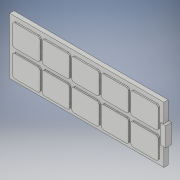
# Autodesk Inventor part: Solar_panel
Saved by Autodesk Inventor 2018 (Build 220112000, 112)
## iProperties
Created: 2021-03-12
Part Number: Solar_panel
Material: Generic
Document SubType Name: Modeling
Designer: Patel
Density: 1 g/cm^3
Appearance: Default
Author: Patel
Autodesk Inventor part; units mm, degrees
ref_plane "YZ Plane" through (0, 0, 0) normal (1, 0, 0) x (0, 1, 0)
ref_plane "XZ Plane" through (0, 0, 0) normal (0, 1, 0) x (-1, 0, 0)
sketch "Sketch1" plane through (0, 0, 0) normal (0, 0, 1) x (1, 0, 0)
  line L0 (-177.5, 65) -> (177.5, 65)
  line L1 (177.5, 65) -> (177.5, -65)
  line L2 (177.5, -65) -> (-177.5, -65)
  line L3 (-177.5, -65) -> (-177.5, 65)
  line L4 (-177.5, 65) -> (177.5, -65) construction
  line L5 (177.5, 65) -> (-177.5, -65) construction
  point P0 (0, 0)
  dimension "d0" = 355
  dimension "d1" = 130
  constraints: 12 end point, 2 midpoint, 2 parallel, 1 horizontal, 1 perpendicular
  measures "d0" distance of L1.end L2.end
  measures "d1" distance of L0.end L1.end
extrude "Extrusion1" add sketch "Sketch1" against normal blind 10
sketch "Sketch2" plane through (0, 0, 0) normal (0, 0, 1) x (1, 0, 0)
  line L0 (-162.5, 55) -> (-109.5, 55)
  line L1 (-104.5, 50) -> (-104.5, 9.1977)
  line L2 (-109.5, 4.1977) -> (-162.5, 4.1977)
  line L3 (-167.5, 9.1977) -> (-167.5, 50)
  line L4 (-177.5, 65) -> (177.5, 65) projected
  line L5 (-177.5, -65) -> (-177.5, 65) projected
  arc A0 (-162.5, 55) -> (-167.5, 50) centre (-162.5, 50) ccw
  arc A1 (-104.5, 50) -> (-109.5, 55) centre (-109.5, 50) ccw
  arc A2 (-109.5, 4.1977) -> (-104.5, 9.1977) centre (-109.5, 9.1977) ccw
  arc A3 (-167.5, 9.1977) -> (-162.5, 4.1977) centre (-162.5, 9.1977) ccw
  line L6 (-94.5, 55) -> (-41.5, 55)
  line L7 (-36.5, 50) -> (-36.5, 9.1977)
  line L8 (-41.5, 4.1977) -> (-94.5, 4.1977)
  line L9 (-99.5, 9.1977) -> (-99.5, 50)
  arc A4 (-94.5, 55) -> (-99.5, 50) centre (-94.5, 50) ccw
  arc A5 (-36.5, 50) -> (-41.5, 55) centre (-41.5, 50) ccw
  arc A6 (-41.5, 4.1977) -> (-36.5, 9.1977) centre (-41.5, 9.1977) ccw
  arc A7 (-99.5, 9.1977) -> (-94.5, 4.1977) centre (-94.5, 9.1977) ccw
  line L10 (-26.5, 55) -> (26.5, 55)
  line L11 (31.5, 50) -> (31.5, 9.1977)
  line L12 (26.5, 4.1977) -> (-26.5, 4.1977)
  line L13 (-31.5, 9.1977) -> (-31.5, 50)
  arc A8 (-26.5, 55) -> (-31.5, 50) centre (-26.5, 50) ccw
  arc A9 (31.5, 50) -> (26.5, 55) centre (26.5, 50) ccw
  arc A10 (26.5, 4.1977) -> (31.5, 9.1977) centre (26.5, 9.1977) ccw
  arc A11 (-31.5, 9.1977) -> (-26.5, 4.1977) centre (-26.5, 9.1977) ccw
  line L14 (41.5, 55) -> (94.5, 55)
  line L15 (99.5, 50) -> (99.5, 9.1977)
  line L16 (94.5, 4.1977) -> (41.5, 4.1977)
  line L17 (36.5, 9.1977) -> (36.5, 50)
  arc A12 (41.5, 55) -> (36.5, 50) centre (41.5, 50) ccw
  arc A13 (99.5, 50) -> (94.5, 55) centre (94.5, 50) ccw
  arc A14 (94.5, 4.1977) -> (99.5, 9.1977) centre (94.5, 9.1977) ccw
  arc A15 (36.5, 9.1977) -> (41.5, 4.1977) centre (41.5, 9.1977) ccw
  line L18 (109.5, 55) -> (162.5, 55)
  line L19 (167.5, 50) -> (167.5, 9.1977)
  line L20 (162.5, 4.1977) -> (109.5, 4.1977)
  line L21 (104.5, 9.1977) -> (104.5, 50)
  arc A16 (109.5, 55) -> (104.5, 50) centre (109.5, 50) ccw
  arc A17 (167.5, 50) -> (162.5, 55) centre (162.5, 50) ccw
  arc A18 (162.5, 4.1977) -> (167.5, 9.1977) centre (162.5, 9.1977) ccw
  arc A19 (104.5, 9.1977) -> (109.5, 4.1977) centre (109.5, 9.1977) ccw
  line L22 (-162.5, -5.802) -> (-109.5, -5.802)
  line L23 (-167.5, -51.6043) -> (-167.5, -10.802)
  line L24 (-109.5, -56.6043) -> (-162.5, -56.6043)
  line L25 (-104.5, -10.802) -> (-104.5, -51.6043)
  line L26 (-99.5, -51.6043) -> (-99.5, -10.802)
  line L27 (-94.5, -5.802) -> (-41.5, -5.802)
  line L28 (-36.5, -10.802) -> (-36.5, -51.6043)
  line L29 (-41.5, -56.6043) -> (-94.5, -56.6043)
  line L30 (-31.5, -51.6043) -> (-31.5, -10.802)
  line L31 (-26.5, -5.802) -> (26.5, -5.802)
  line L32 (31.5, -10.802) -> (31.5, -51.6043)
  line L33 (26.5, -56.6043) -> (-26.5, -56.6043)
  line L34 (41.5, -5.802) -> (94.5, -5.802)
  line L35 (36.5, -51.6043) -> (36.5, -10.802)
  line L36 (94.5, -56.6043) -> (41.5, -56.6043)
  line L37 (99.5, -10.802) -> (99.5, -51.6043)
  line L38 (104.5, -51.6043) -> (104.5, -10.802)
  line L39 (109.5, -5.802) -> (162.5, -5.802)
  line L40 (167.5, -10.802) -> (167.5, -51.6043)
  line L41 (162.5, -56.6043) -> (109.5, -56.6043)
  arc A20 (-162.5, -5.802) -> (-167.5, -10.802) centre (-162.5, -10.802) ccw
  arc A21 (-104.5, -10.802) -> (-109.5, -5.802) centre (-109.5, -10.802) ccw
  arc A22 (-167.5, -51.6043) -> (-162.5, -56.6043) centre (-162.5, -51.6043) ccw
  arc A23 (-109.5, -56.6043) -> (-104.5, -51.6043) centre (-109.5, -51.6043) ccw
  arc A24 (-99.5, -51.6043) -> (-94.5, -56.6043) centre (-94.5, -51.6043) ccw
  arc A25 (-94.5, -5.802) -> (-99.5, -10.802) centre (-94.5, -10.802) ccw
  arc A26 (-36.5, -10.802) -> (-41.5, -5.802) centre (-41.5, -10.802) ccw
  arc A27 (-26.5, -5.802) -> (-31.5, -10.802) centre (-26.5, -10.802) ccw
  arc A28 (-41.5, -56.6043) -> (-36.5, -51.6043) centre (-41.5, -51.6043) ccw
  arc A29 (-31.5, -51.6043) -> (-26.5, -56.6043) centre (-26.5, -51.6043) ccw
  arc A30 (31.5, -10.802) -> (26.5, -5.802) centre (26.5, -10.802) ccw
  arc A31 (26.5, -56.6043) -> (31.5, -51.6043) centre (26.5, -51.6043) ccw
  arc A32 (36.5, -51.6043) -> (41.5, -56.6043) centre (41.5, -51.6043) ccw
  arc A33 (41.5, -5.802) -> (36.5, -10.802) centre (41.5, -10.802) ccw
  arc A34 (99.5, -10.802) -> (94.5, -5.802) centre (94.5, -10.802) ccw
  arc A35 (94.5, -56.6043) -> (99.5, -51.6043) centre (94.5, -51.6043) ccw
  arc A36 (104.5, -51.6043) -> (109.5, -56.6043) centre (109.5, -51.6043) ccw
  arc A37 (109.5, -5.802) -> (104.5, -10.802) centre (109.5, -10.802) ccw
  arc A38 (167.5, -10.802) -> (162.5, -5.802) centre (162.5, -10.802) ccw
  arc A39 (162.5, -56.6043) -> (167.5, -51.6043) centre (162.5, -51.6043) ccw
  line L42 (171.5, 22) -> (183.5, 22)
  line L43 (183.5, 22) -> (183.5, -22)
  line L44 (183.5, -22) -> (171.5, -22)
  line L45 (171.5, -22) -> (171.5, 22)
  line L46 (177.5, 65) -> (177.5, -65) projected
  line L47 (171.5, 22) -> (183.5, -22) construction
  line L48 (183.5, 22) -> (171.5, -22) construction
  point P0 (0, 0)
  point P1 (-167.5, 55)
  point P2 (-104.5, 55)
  point P3 (-167.5, 4.1977)
  point P4 (-99.5, 55)
  point P5 (-36.5, 55)
  point P6 (-99.5, 4.1977)
  point P7 (-31.5, 55)
  point P8 (31.5, 55)
  point P9 (-31.5, 4.1977)
  point P10 (36.5, 55)
  point P11 (99.5, 55)
  point P12 (36.5, 4.1977)
  point P13 (104.5, 55)
  point P14 (167.5, 55)
  point P15 (104.5, 4.1977)
  point P16 (-167.5, -5.802)
  point P17 (-104.5, -5.802)
  point P18 (-167.5, -56.6043)
  point P19 (-99.5, -5.802)
  point P20 (-99.5, -56.6043)
  point P21 (-36.5, -5.802)
  point P22 (-31.5, -5.802)
  point P23 (-31.5, -56.6043)
  point P24 (31.5, -5.802)
  point P25 (36.5, -5.802)
  point P26 (99.5, -5.802)
  point P27 (36.5, -56.6043)
  point P28 (104.5, -5.802)
  point P29 (104.5, -56.6043)
  point P30 (167.5, -5.802)
  point P31 (177.5, 0)
  dimension "d4" = 10
  dimension "d5" = 10
  dimension "d7" = 50.8023
  dimension "d8" = 63
  dimension "d9" = 5
  dimension "d12" = 68
  dimension "d19" = 60.802
  dimension "d24" = 12
  dimension "d25" = 44
  constraints: 92 end point, 80 point on circle, 60 point on line, 40 centre point, 8 tangent, 4 parallel, 3 equal radius, 3 horizontal, 3 midpoint, 2 perpendicular, 1 vertical, 207 other
  measures "d4" distance between parallel lines of L4 L0
  measures "d5" distance between parallel lines of L5 L3
  measures "d7" distance of point (-167.5, 4.198) point (-167.5, 55)
  measures "d8" distance of point (-167.5, 55) point (-104.5, 55)
  measures "d9" radius of A0
  measures "d12" distance of L0.start L6.start
  measures "d19" distance of L0.start L22.start
  measures "d24" distance of L43.end L44.end
  measures "d25" distance of L42.end L43.end
extrude "Extrusion2" add sketch "Sketch2" along normal blind 3 contours L0 A1 L1 A2 L2 A3 L3 A0 | L6 A5 L7 A6 L8 A7 L9 A4 | L10 A9 L11 A10 L12 A11 L13 A8 | L14 A13 L15 A14 L16 A15 L17 A12 | L18 A17 L19 A18 L20 A19 L21 A16 | L22 A21 L25 A23 L24 A22 L23 A20 | L26 A25 L27 A26 L28 A28 L29 A24 | L30 A27 L31 A30 L32 A31 L33 A29 | L34 A34 L37 A35 L36 A32 L35 A33 | L38 A37 L39 A38 L40 A39 L41 A36
ref_plane "Work Plane1" through (0, 0, -5) normal (0, 0, 1) x (1, 0, 0)
sketch "Sketch3" plane through (0, 0, -5) normal (0, 0, 1) x (1, 0, 0)
  line L0 (171.5, 22) -> (183.5, 22)
  line L1 (183.5, 22) -> (183.5, -22)
  line L2 (183.5, -22) -> (171.5, -22)
  line L3 (171.5, -22) -> (171.5, 22)
  line L4 (177.5, 65) -> (177.5, -65) projected
  line L5 (171.5, 22) -> (183.5, -22) construction
  line L6 (183.5, 22) -> (171.5, -22) construction
  point P0 (0, 0)
  point P1 (177.5, 0)
  dimension "d31" = 12
  dimension "d32" = 44
  constraints: 12 end point, 3 midpoint, 2 parallel, 1 horizontal, 1 perpendicular
  measures "d31" distance of L1.end L2.end
  measures "d32" distance of L0.end L1.end
extrude "Extrusion3" add sketch "Sketch3" along normal mid plane 14
body "Solid1"
